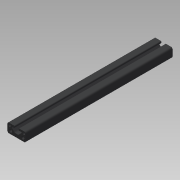
# Autodesk Inventor part: 1575
Saved by Autodesk Inventor 2013 (Build 170138000, 138)
## iProperties
Company: 80/20 Inc.
Created: 2014-04-23
Part Number: 1575
Material: Generic
Document SubType Name: Modeling
Density: 1 g/cm^3
Vendor: 80/20 Inc.
Engineer: Ross Bowman
Designer: Ross Bowman
Catalog Web Link: 8020.net
Material: 6105-T5 Aluminum
Author: Ross Bowman
Keywords: 80/20 , 8020 , T-Slot , Extrusion
Autodesk Inventor part; units mm, degrees
ref_plane "YZ Plane" through (0, 0, 0) normal (1, 0, 0) x (0, 1, 0)
ref_plane "XZ Plane" through (0, 0, 0) normal (0, 1, 0) x (-1, 0, 0)
ref_plane "XY Plane" through (0, 0, 0) normal (0, 0, 1) x (1, 0, 0)
sketch "Sketch1" plane through (0, 0, 0) normal (0, 0, 1) x (1, 0, 0)
  circle A0 centre (14.8488, 5.2764) radius 2.5527
  circle A1 centre (12.7, -3.175) radius 3.3274
  circle A2 centre (-12.7, -3.175) radius 3.3274
  circle A3 centre (-14.8488, 5.2764) radius 2.5527
  arc A4 (-9.398, 5.461) -> (-10.287, 4.572) centre (-9.398, 4.572) ccw
  line L0 (-9.398, 5.461) -> (-5.334, 5.461)
  arc A5 (-5.334, 5.461) -> (-4.064, 6.731) centre (-5.334, 6.731) ccw
  line L1 (-4.064, 6.731) -> (-4.064, 8.001)
  arc A6 (-4.064, 8.001) -> (-5.588, 9.525) centre (-5.588, 8.001) ccw
  line L2 (-5.588, 9.525) -> (-15.875, 9.525)
  arc A7 (-15.875, 9.525) -> (-19.05, 6.35) centre (-15.875, 6.35) ccw
  line L3 (-19.05, 6.35) -> (-19.05, -6.35)
  arc A8 (-19.05, -6.35) -> (-15.875, -9.525) centre (-15.875, -6.35) ccw
  line L4 (-15.875, -9.525) -> (15.875, -9.525)
  arc A9 (15.875, -9.525) -> (19.05, -6.35) centre (15.875, -6.35) ccw
  line L5 (19.05, -6.35) -> (19.05, 6.35)
  arc A10 (19.05, 6.35) -> (15.875, 9.525) centre (15.875, 6.35) ccw
  line L6 (15.875, 9.525) -> (5.588, 9.525)
  arc A11 (5.588, 9.525) -> (4.064, 8.001) centre (5.588, 8.001) ccw
  line L7 (4.064, 8.001) -> (4.064, 6.731)
  arc A12 (4.064, 6.731) -> (5.334, 5.461) centre (5.334, 6.731) ccw
  line L8 (5.334, 5.461) -> (9.398, 5.461)
  arc A13 (10.287, 4.572) -> (9.398, 5.461) centre (9.398, 4.572) ccw
  line L9 (10.287, 4.572) -> (10.287, 4.2554)
  arc A14 (10.0266, 3.6267) -> (10.287, 4.2554) centre (9.398, 4.2554) ccw
  line L10 (10.0266, 3.6267) -> (5.1241, -1.2758)
  arc A15 (1.7654, -2.667) -> (5.1241, -1.2758) centre (1.7654, 2.0828) ccw
  line L11 (1.7654, -2.667) -> (-1.7654, -2.667)
  arc A16 (-5.1241, -1.2758) -> (-1.7654, -2.667) centre (-1.7654, 2.0828) ccw
  line L12 (-5.1241, -1.2758) -> (-10.0266, 3.6267)
  arc A17 (-10.287, 4.2554) -> (-10.0266, 3.6267) centre (-9.398, 4.2554) ccw
  line L13 (-10.287, 4.2554) -> (-10.287, 4.572)
  point P0 (0, 0)
  constraints: 28 end point, 28 point on circle, 18 centre point
extrude "Extrusion1" add sketch "Sketch1" against normal blind 304.8
body "Solid1"
